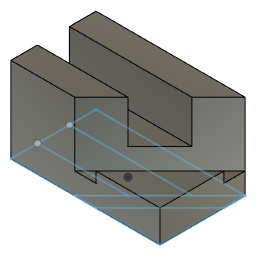
ex63 (Autodesk Fusion 360 design; units mm, degrees)
Autodesk Fusion 360 part; units mm, degrees
sketch "Sketch1" plane through (0, 0, 0) normal (0, 0, 1) x (1, 0, 0)
  line L0 (35, 20) -> (-35, 20)
  line L1 (-35, 20) -> (-35, -20)
  line L2 (-35, -20) -> (35, -20)
  line L3 (35, -20) -> (35, 20)
  line L4 (0, -20) -> (-5, -20)
  line L5 (0, -20) -> (5, -20)
  line L6 (35, 20) -> (35, 15)
  line L7 (35, 15) -> (35, 10)
  line L8 (35, 10) -> (5, -20)
  line L9 (35, 20) -> (-5, -20)
  line L10 (-35, -7.5) -> (7.5, -7.5)
  line L11 (-35, 7.5) -> (22.5, 7.5)
  dimension "d8" = 70
  dimension "d9" = 40
  dimension "d14" = 5
  dimension "d15" = 5
  dimension "d16" = 5
  dimension "d17" = 5
  constraint horizontal L0
  constraint perpendicular L0 L1
  constraint parallel L0 L2
  constraint parallel L1 L3
  constraint midpoint L2 L4.start
  constraint perpendicular L0 L6
  constraint parallel L3 L7
  constraint coincident L9 L10.end
  constraint coincident L9 L11.end
  measures "d8" distance of L1.end L2.end
  measures "d9" distance of L0.end L1.end
  measures "d14" distance of L4.start L4.end
  measures "d15" distance of L4.start L5.end
  measures "d16" distance of L0.start L6.end
  measures "d17" distance of L6.end L7.end
extrude "Extrude1" add sketch "Sketch1" along normal blind 10 contours L2 L3 L4 L5 L6 L7 L8 L9
extrude "Extrude2" add sketch "Sketch1" along normal blind 40 contours L0 L1 L9 L11 | L1 L2 L9 L10
extrude "Extrude3" add sketch "Sketch1" along normal blind 15 contours L2 L3 L8
extrude "Extrude4" add sketch "Sketch1" along normal blind 20 contours L1 L9 L10 L11
